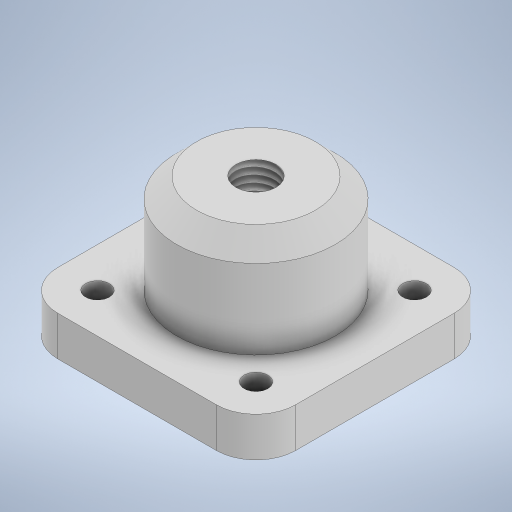
# Autodesk Inventor part: Valve Bonnet
Saved by Autodesk Inventor 2023 (Build 270158030, 158C)
## iProperties
Created: 2022-11-22
Part Number: Valve Bonnet
Material: Generic
Document SubType Name: Modeling
Designer: Imogen Heard
Density: 1 g/cm^3
Appearance: Default
Author: Imogen Heard
Autodesk Inventor part; units mm, degrees
ref_plane "YZ Plane" through (0, 0, 0) normal (1, 0, 0) x (0, 1, 0)
ref_plane "XZ Plane" through (0, 0, 0) normal (0, 1, 0) x (-1, 0, 0)
ref_plane "XY Plane" through (0, 0, 0) normal (0, 0, 1) x (1, 0, 0)
sketch "Sketch1" plane through (0, 0, 0) normal (0, 1, 0) x (-1, 0, 0)
  line L0 (-10, -60) -> (-50, -60)
  line L1 (-60, -50) -> (-60, -10)
  line L2 (-50, 0) -> (-10, 0)
  line L3 (0, -10) -> (0, -50)
  arc A0 (-60, -50) -> (-50, -60) centre (-50, -50) ccw
  arc A1 (-10, -60) -> (0, -50) centre (-10, -50) ccw
  arc A2 (0, -10) -> (-10, 0) centre (-10, -10) ccw
  arc A3 (-50, 0) -> (-60, -10) centre (-50, -10) ccw
  circle A4 centre (-10, -50) radius 3
  circle A5 centre (-50, -50) radius 3
  circle A6 centre (-10, -10) radius 3
  circle A7 centre (-50, -10) radius 3
  point P0 (0, 0)
  point P1 (0, 0)
  point P2 (-30, 0)
  dimension "d0" = 60
  dimension "d1" = 60
  dimension "d2" = 10
  dimension "d3" = 6
  constraints: 8 centre point, 8 end point, 8 point on circle, 8 tangent, 6 equal radius, 4 concentric, 2 parallel, 2 point on line, 1 coincident, 1 horizontal, 1 midpoint, 1 perpendicular
  measures "d0" distance between parallel lines of L1 L3
  measures "d1" distance from line of point (-30, 0) L0
  measures "d2" radius of A0
  measures "d3" diameter of A4
extrude "Extrusion1" add sketch "Sketch1" along normal blind 10
sketch "Sketch2" plane through (0, 10, 0) normal (0, 1, 0) x (1, 0, 0)
  line L0 (0, 50) -> (0, 10) projected
  line L1 (0, 30) -> (60, 30)
  line L2 (60, 10) -> (60, 50) projected
  line L3 (30, 60) -> (30, 0)
  line L4 (10, 0) -> (50, 0) projected
  line L5 (50, 60) -> (10, 60) projected
  circle A0 centre (30, 30) radius 20
  point P0 (0, 0)
  point P1 (30, 0)
  dimension "d6" = 40
  constraints: 6 midpoint, 4 coincident, 4 end point, 1 centre point, 1 vertical
  measures "d6" diameter of A0
extrude "Extrusion2" add sketch "Sketch2" along normal blind 25
chamfer "Chamfer1" distance 5 angle 45 1 edges at (10, 35, -30)
sketch "Sketch3" plane through (0, 0, 0) normal (0, -1, 0) x (1, 0, 0)
  circle A0 centre (30, -30) radius 15 projected
  point P0 (0, 0)
extrude "Extrusion3" cut sketch "Sketch3" against normal blind 20
sketch "Sketch4" plane through (0, 0, 0) normal (0, -1, 0) x (1, 0, 0)
  circle A0 centre (30, -30) radius 20 projected
  point P0 (0, 0)
extrude "Extrusion4" cut sketch "Sketch4" against normal blind 5
sketch "Sketch5" plane through (30, 35, -30) normal (0, 1, 0) x (1, 0, 0)
  circle A0 centre (0, 0) radius 6
  circle A1 centre (0, 0) radius 15 projected
  point P0 (-30, -30)
  dimension "d16" = 12
  constraints: 1 centre point, 1 concentric
  measures "d16" diameter of A0
hole "Hole1" at (30, 35, -30) direction (0, -1, 0) diameter 10.106 end through all thread size "M12x1.75" class "6H" standard "ISO Metric profile"
body "Solid1"
